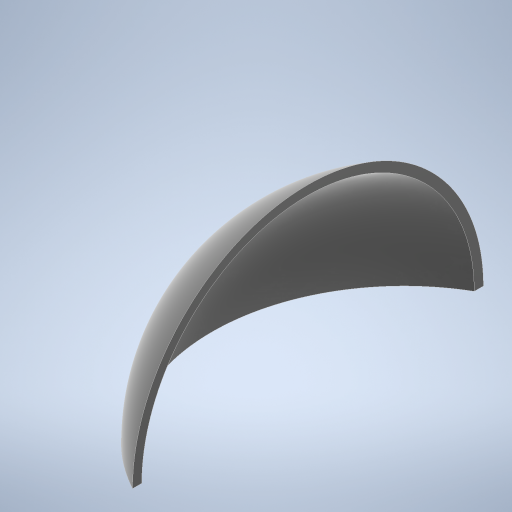
# Autodesk Inventor part: Part11
Saved by Autodesk Inventor 2023 (Build 270158000, 158)
## iProperties
Created: 2022-11-23
Part Number: Part11
Material: PC/ABS プラスチック
Document SubType Name: Modeling
Designer: yuta
Density: 0.357273 g/cm^3
Appearance: 滑らか - 黒
Author: yuta
Autodesk Inventor part; units mm, degrees
ref_plane "YZ Plane" through (0, 0, 0) normal (1, 0, 0) x (0, 1, 0)
ref_plane "XZ Plane" through (0, 0, 0) normal (0, 1, 0) x (-1, 0, 0)
ref_plane "XY Plane" through (0, 0, 0) normal (0, 0, 1) x (1, 0, 0)
sketch "スケッチ1" plane through (0, 0, 0) normal (0, 0, 1) x (1, 0, 0)
  arc A0 (0, 125) -> (-125, 0) centre (0, 0) ccw
  line L0 (0, 125) -> (0, 0)
  line L1 (0, 0) -> (-125, 0)
  point P0 (0, 0)
  dimension "d0" = 125
  dimension "d1" = 125
  dimension "d2" = 125
  constraints: 4 end point, 2 point on circle, 1 centre point, 1 perpendicular, 1 vertical
  measures "d0" distance of point (0, 0) L1.end
  measures "d1" distance of point (0, 0) L0.start
  measures "d2" radius of A0
revolve "回転1" add sketch "スケッチ1" angle 360 about axis through (0, 125, 0) along (0, -1, 0)
sketch "スケッチ2" plane through (0, 0, 0) normal (0, -1, 0) x (1, 0, 0)
  line L0 (60, -130) -> (-60, -130)
  line L1 (-60, -130) -> (-60, 130)
  line L2 (-60, 130) -> (60, 130)
  line L3 (60, 130) -> (60, -130)
  line L4 (60, -130) -> (-60, 130) construction
  line L5 (-60, -130) -> (60, 130) construction
  line L6 (177.9877, -390) -> (60, -390)
  line L7 (60, -390) -> (60, 130)
  line L8 (60, 130) -> (177.9877, 130)
  line L9 (177.9877, 130) -> (177.9877, -390)
  line L10 (177.9877, -390) -> (60, 130) construction
  line L11 (60, -390) -> (177.9877, 130) construction
  point P0 (0, 0)
  point P1 (118.9938, -130)
  dimension "d4" = 120
  dimension "d5" = 260
  constraints: 24 end point, 4 midpoint, 4 parallel, 2 horizontal, 2 perpendicular, 1 point on line
  measures "d4" distance of L1.end L2.end
  measures "d5" distance of L0.end L1.end
extrude "押し出し1" cut sketch "スケッチ2" against normal blind 200
sketch "スケッチ3" plane through (0, 0, 0) normal (0, -1, 0) x (1, 0, 0)
  circle A0 centre (0, 0) radius 120
  line L0 (0, 0) -> (0, 7.6881)
  line L1 (0, 120) -> (0, -120)
  dimension "d8" = 240
  constraints: 4 end point, 2 point on circle, 2 vertical, 1 centre point, 1 coincident
  measures "d8" diameter of A0
revolve "回転2" cut sketch "スケッチ3" angle 360 about axis through (0, 0, 120) along (0, 0, -1) picked at (-69.9662, -38.4642) contours L1 L0 A0
